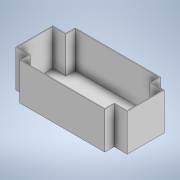
# Autodesk Inventor part: Footprint
Saved by Autodesk Inventor 2021 (Build 250183000, 183)
## iProperties
Created: 2020-11-11
Part Number: Footprint
Material: Generic
Document SubType Name: Modeling
Designer: coupe
Density: 1 g/cm^3
Appearance: Default
Mass: 104.423 g
Surface Area: 544.305 cm^2
Volume: 104.423 cm^3
Author: coupe
Autodesk Inventor part; units mm, degrees
ref_plane "YZ Plane" through (0, 0, 0) normal (1, 0, 0) x (0, 1, 0)
ref_plane "XZ Plane" through (0, 0, 0) normal (0, 1, 0) x (-1, 0, 0)
sketch "Sketch1" plane through (0, 0, 0) normal (0, 0, 1) x (1, 0, 0)
  line L0 (0, 0) -> (152.4, 0)
  line L1 (152.4, 0) -> (152.4, 50.8)
  line L2 (152.4, 50.8) -> (0, 50.8)
  line L3 (0, 50.8) -> (0, 0)
  line L4 (0, 50.8) -> (17.78, 50.8)
  line L5 (17.78, 0) -> (0, 0)
  line L6 (0, 0) -> (0, 50.8)
  line L7 (152.4, 0) -> (134.62, 0)
  line L8 (134.62, 50.8) -> (152.4, 50.8)
  line L9 (152.4, 50.8) -> (152.4, 0)
  dimension "d0" = 152.4
  dimension "d1" = 50.8
  constraints: 20 end point, 4 parallel, 3 horizontal, 2 point on line, 1 perpendicular
  measures "d0" distance between parallel lines of L3 L1
  measures "d1" distance between parallel lines of L0 L2
extrude "Extrusion1" add sketch "Sketch1" against normal blind 38.1
sketch "Sketch2" plane through (0, 0, 0) normal (0, 0, 1) x (1, 0, 0)
  line L0 (0, 50.8) -> (152.4, 50.8) projected
  line L1 (152.4, 0) -> (0, 0) projected
  line L2 (0, 50.8) -> (17.78, 50.8)
  line L3 (17.78, 50.8) -> (17.78, 0)
  line L4 (17.78, 0) -> (0, 0)
  line L5 (0, 0) -> (0, 50.8)
  line L6 (152.4, 0) -> (134.62, 0)
  line L7 (134.62, 0) -> (134.62, 50.8)
  line L8 (134.62, 50.8) -> (152.4, 50.8)
  line L9 (152.4, 50.8) -> (152.4, 0)
  point P0 (134.62, 0)
  dimension "d6" = 17.78
  dimension "d7" = 17.78
  constraints: 16 end point, 4 parallel, 2 horizontal, 2 perpendicular, 2 point on line
  measures "d6" distance between parallel lines of L5 L3
  measures "d7" distance between parallel lines of L9 L7
extrude "Extrusion2" cut sketch "Sketch2" against normal blind 12.8 contours L0 L3 L1 L5 | L0 L9 L1 L7
shell "Shell1" thickness 1 removed faces 2 at (56.7267, 50.8, -29.6667) at (101.6, 16.9333, -38.1)
ref_plane "Work Plane3" through (133.62, 1, -38.1) normal (0, 0, -1) x (-1, 0, 0)
mirror "Mirror2" about plane through (133.62, 1, -38.1) normal (0, 0, -1) of "Extrusion1", "Extrusion2"
shell "Shell6" thickness 1 removed faces 2 at (95.6733, 50.8, -46.5333) at (101.2667, 17.6, -38.1)
body "Solid1"
